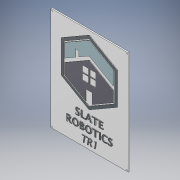
# Autodesk Inventor part: BP002b
Saved by Autodesk Inventor 2017 SP1 (Build 210196100, 196)
## iProperties
Created: 2017-12-18
Part Number: BP002b
Material: ABS Plastic
Document SubType Name: Modeling
Designer: Zach
Density: 1.06 g/cm^3
Appearance: CR White
Author: Zach
Autodesk Inventor part; units mm, degrees
ref_plane "YZ Plane" through (0, 0, 0) normal (1, 0, 0) x (0, 1, 0)
ref_plane "XZ Plane" through (0, 0, 0) normal (0, 1, 0) x (-1, 0, 0)
ref_plane "XY Plane" through (0, 0, 0) normal (0, 0, 1) x (1, 0, 0)
sketch "Sketch1" plane through (0, 0, 0) normal (0, 0, 1) x (1, 0, 0)
  line L0 (0, 0) -> (300, 0)
  line L1 (300, 0) -> (300, 400)
  line L2 (300, 400) -> (0, 400)
  line L3 (0, 400) -> (0, 0)
  line L4 (5, 5) -> (295, 5) construction
  line L5 (295, 5) -> (295, 395) construction
  line L6 (295, 395) -> (5, 395) construction
  line L7 (5, 395) -> (5, 5) construction
  circle A0 centre (5, 395) radius 2.5
  circle A1 centre (295, 395) radius 2.5
  circle A2 centre (295, 5) radius 2.5
  circle A3 centre (5, 5) radius 2.5
  dimension "d0" = 300
  dimension "d1" = 400
  dimension "d2" = 5
  dimension "d3" = 5
  dimension "d4" = 5
  dimension "d5" = 5
  dimension "d6" = 5
  constraints: 16 end point, 4 centre point, 4 coincident, 4 parallel, 2 perpendicular, 1 horizontal, 3 other
  measures "d0" distance of L2.end L1.end
  measures "d1" distance of L1.end L0.end
  measures "d2" distance between parallel lines of L3 L7
  measures "d3" diameter of A0
  measures "d4" diameter of A1
  measures "d5" diameter of A2
  measures "d6" diameter of A3
extrude "Extrusion1" add sketch "Sketch1" along normal blind 5
sketch "Sketch2" plane through (0, 0, 5) normal (0, 0, 1) x (1, 0, 0)
  line L0 (0, 135) -> (300, 135) construction
  line L1 (300, 135) -> (300, 0) construction
  line L2 (300, 0) -> (0, 0) construction
  line L3 (0, 0) -> (0, 135) construction
  line L4 (25, 385) -> (275, 385) construction
  line L5 (275, 385) -> (275, 135) construction
  line L6 (275, 135) -> (25, 135) construction
  line L7 (25, 135) -> (25, 385) construction
  line L8 (300, 400) -> (0, 400) projected
  line L9 (300, 0) -> (300, 400) projected
  line L10 (150, 385) -> (258.2532, 322.5)
  line L11 (258.2532, 322.5) -> (258.2532, 197.5)
  line L12 (258.2532, 197.5) -> (150, 135)
  line L13 (150, 135) -> (41.7468, 197.5)
  line L14 (41.7468, 197.5) -> (41.7468, 322.5)
  line L15 (41.7468, 322.5) -> (150, 385)
  line L16 (150, 373.2221) -> (248.0532, 316.611)
  line L17 (248.0532, 316.611) -> (248.0532, 203.389)
  line L18 (248.0532, 203.389) -> (150, 146.7779)
  line L19 (150, 146.7779) -> (51.9468, 203.389)
  line L20 (51.9468, 203.389) -> (51.9468, 316.611)
  line L21 (51.9468, 316.611) -> (150, 373.2221)
  line L22 (150, 368.3146) -> (243.8032, 314.1573) construction
  line L23 (243.8032, 314.1573) -> (243.8032, 205.8427) construction
  line L24 (243.8032, 205.8427) -> (150, 151.6854) construction
  line L25 (150, 151.6854) -> (56.1968, 205.8427) construction
  line L26 (56.1968, 205.8427) -> (56.1968, 314.1573) construction
  line L27 (56.1968, 314.1573) -> (150, 368.3146) construction
  line L28 (56.1968, 261.6573) -> (96.1968, 284.7513)
  line L29 (96.1968, 284.7513) -> (96.1968, 313.2513)
  line L30 (96.1968, 313.2513) -> (110.1968, 313.2513)
  line L31 (110.1968, 313.2513) -> (110.1968, 292.8342)
  line L32 (110.1968, 292.8342) -> (150, 315.8146)
  line L33 (150, 315.8146) -> (243.8032, 261.6573)
  line L34 (243.8032, 261.6573) -> (243.8032, 314.1573)
  line L35 (243.8032, 314.1573) -> (150, 368.3146)
  line L36 (150, 368.3146) -> (56.1968, 314.1573)
  line L37 (56.1968, 261.6573) -> (56.1968, 314.1573)
  line L38 (56.1968, 205.8427) -> (138, 158.6136)
  line L39 (138, 158.6136) -> (138, 198.6854)
  line L40 (138, 198.6854) -> (162, 198.6854)
  line L41 (162, 198.6854) -> (162, 158.6136)
  line L42 (162, 158.6136) -> (243.8032, 205.8427)
  line L43 (243.8032, 205.8427) -> (243.8032, 246.6573)
  line L44 (243.8032, 246.6573) -> (150, 300.8146)
  line L45 (150, 300.8146) -> (56.1968, 246.6573)
  line L46 (56.1968, 246.6573) -> (56.1968, 205.8427)
  line L47 (123.75, 272.6854) -> (176.25, 272.6854) construction
  line L48 (176.25, 272.6854) -> (176.25, 221.6854) construction
  line L49 (176.25, 221.6854) -> (123.75, 221.6854) construction
  line L50 (123.75, 221.6854) -> (123.75, 272.6854) construction
  line L51 (123.75, 221.6854) -> (147.75, 221.6854)
  line L52 (147.75, 221.6854) -> (147.75, 245.6854)
  line L53 (147.75, 245.6854) -> (123.75, 245.6854)
  line L54 (123.75, 245.6854) -> (123.75, 221.6854)
  line L55 (123.75, 272.6854) -> (147.75, 272.6854)
  line L56 (147.75, 272.6854) -> (147.75, 248.6854)
  line L57 (147.75, 248.6854) -> (123.75, 248.6854)
  line L58 (123.75, 248.6854) -> (123.75, 272.6854)
  line L59 (176.25, 272.6854) -> (152.25, 272.6854)
  line L60 (152.25, 272.6854) -> (152.25, 248.6854)
  line L61 (152.25, 248.6854) -> (176.25, 248.6854)
  line L62 (176.25, 248.6854) -> (176.25, 272.6854)
  line L63 (176.25, 221.6854) -> (152.25, 221.6854)
  line L64 (152.25, 221.6854) -> (152.25, 245.6854)
  line L65 (152.25, 245.6854) -> (176.25, 245.6854)
  line L66 (176.25, 245.6854) -> (176.25, 221.6854)
  line L67 (96.7483, 94.8958) -> (96.7483, 99.1804)
  spline S0 degree 2 poles (96.7483, 99.1804) (99.6748, 97.9563) (102.5631, 97.4781) (103.7682, 97.4781) knots 0 0 0 1 2 2 2
  spline S1 degree 2 poles (103.7682, 97.4781) (105.9487, 97.4781) (108.1102, 99.4291) (108.1102, 100.8063) knots 0 0 0 1 2 2 2
  spline S2 degree 2 poles (108.1102, 100.8063) (108.1102, 101.8583) (107.5172, 102.7) knots 0 0 0 1 1 1
  spline S3 degree 2 poles (107.5172, 102.7) (106.9051, 103.5224) (104.5524, 104.8423) knots 0 0 0 1 1 1
  line L68 (104.5524, 104.8423) -> (102.8692, 105.7795)
  spline S4 degree 2 poles (102.8692, 105.7795) (99.254, 107.7879) (97.9916, 109.4903) knots 0 0 0 1 1 1
  spline S5 degree 2 poles (97.9916, 109.4903) (96.6909, 111.1927) (96.6909, 113.4306) knots 0 0 0 1 1 1
  spline S6 degree 2 poles (96.6909, 113.4306) (96.6909, 116.2615) (101.0138, 120.2784) (105.0497, 120.2784) knots 0 0 0 1 2 2 2
  spline S7 degree 2 poles (105.0497, 120.2784) (108.0719, 120.2784) (111.8592, 119.4176) knots 0 0 0 1 1 1
  line L69 (111.8592, 119.4176) -> (111.8592, 115.4199)
  spline S8 degree 2 poles (111.8592, 115.4199) (107.9763, 116.8545) (105.7001, 116.8545) knots 0 0 0 1 1 1
  spline S9 degree 2 poles (105.7001, 116.8545) (103.8064, 116.8545) (101.8363, 115.2095) (101.8363, 114.0618) knots 0 0 0 1 2 2 2
  spline S10 degree 2 poles (101.8363, 114.0618) (101.8363, 113.182) (102.4484, 112.436) knots 0 0 0 1 1 1
  spline S11 degree 2 poles (102.4484, 112.436) (103.0222, 111.6709) (105.3749, 110.3511) knots 0 0 0 1 1 1
  line L70 (105.3749, 110.3511) -> (107.1729, 109.3564)
  spline S12 degree 2 poles (107.1729, 109.3564) (111.3236, 107.042) (112.4522, 105.3396) knots 0 0 0 1 1 1
  spline S13 degree 2 poles (112.4522, 105.3396) (113.5807, 103.6181) (113.5807, 101.4758) knots 0 0 0 1 1 1
  spline S14 degree 2 poles (113.5807, 101.4758) (113.5807, 98.3962) (108.8944, 94.0542) (103.7873, 94.0542) knots 0 0 0 1 2 2 2
  spline S15 degree 2 poles (103.7873, 94.0542) (100.7651, 94.0542) (96.7483, 94.8958) knots 0 0 0 1 1 1
  line L71 (117.9036, 94.6663) -> (117.9036, 119.6663)
  line L72 (117.9036, 119.6663) -> (123.1064, 119.6663)
  line L73 (123.1064, 119.6663) -> (123.1064, 98.2049)
  line L74 (123.1064, 98.2049) -> (134.2578, 98.2049)
  line L75 (134.2578, 98.2049) -> (134.2578, 94.6663)
  line L76 (134.2578, 94.6663) -> (117.9036, 94.6663)
  line L77 (135.2716, 94.6663) -> (144.9694, 119.6663)
  line L78 (144.9694, 119.6663) -> (150.1913, 119.6663)
  line L79 (150.1913, 119.6663) -> (159.9273, 94.6663)
  line L80 (159.9273, 94.6663) -> (154.5907, 94.6663)
  line L81 (154.5907, 94.6663) -> (151.9893, 101.3419)
  line L82 (151.9893, 101.3419) -> (141.6603, 101.3419)
  line L83 (141.6603, 101.3419) -> (139.0589, 94.6663)
  line L84 (139.0589, 94.6663) -> (135.2716, 94.6663)
  line L85 (142.9419, 104.6701) -> (150.6886, 104.6701)
  line L86 (150.6886, 104.6701) -> (146.8248, 114.6357)
  line L87 (146.8248, 114.6357) -> (142.9419, 104.6701)
  line L88 (169.6825, 94.6663) -> (169.6825, 116.2233)
  line L89 (169.6825, 116.2233) -> (160.7307, 116.2233)
  line L90 (160.7307, 116.2233) -> (160.7307, 119.6663)
  line L91 (160.7307, 119.6663) -> (183.837, 119.6663)
  line L92 (183.837, 119.6663) -> (183.837, 116.2233)
  line L93 (183.837, 116.2233) -> (174.8852, 116.2233)
  line L94 (174.8852, 116.2233) -> (174.8852, 94.6663)
  line L95 (174.8852, 94.6663) -> (169.6825, 94.6663)
  line L96 (187.3183, 94.6663) -> (187.3183, 119.6663)
  line L97 (187.3183, 119.6663) -> (203.3282, 119.6663)
  line L98 (203.3282, 119.6663) -> (203.3282, 116.2233)
  line L99 (203.3282, 116.2233) -> (192.521, 116.2233)
  line L100 (192.521, 116.2233) -> (192.521, 109.2608)
  line L101 (192.521, 109.2608) -> (201.4537, 109.2608)
  line L102 (201.4537, 109.2608) -> (201.4537, 105.8178)
  line L103 (201.4537, 105.8178) -> (192.521, 105.8178)
  line L104 (192.521, 105.8178) -> (192.521, 98.2049)
  line L105 (192.521, 98.2049) -> (204.1316, 98.2049)
  line L106 (204.1316, 98.2049) -> (204.1316, 94.6663)
  line L107 (204.1316, 94.6663) -> (187.3183, 94.6663)
  line L108 (61.9836, 54.7098) -> (61.9836, 79.7098)
  line L109 (61.9836, 79.7098) -> (71.337, 79.7098)
  spline S16 degree 2 poles (71.337, 79.7098) (74.2062, 79.7098) (77.2093, 78.2752) (78.9499, 75.3486) (78.9499, 73.5124) knots 0 0 0 1 2 3 3 3
  spline S17 degree 2 poles (78.9499, 73.5124) (78.9499, 71.3127) (76.425, 67.4106) (74.1106, 66.3777) knots 0 0 0 1 2 2 2
  line L110 (74.1106, 66.3777) -> (82.2781, 54.7098)
  line L111 (82.2781, 54.7098) -> (75.9468, 54.7098)
  line L112 (75.9468, 54.7098) -> (69.7303, 64.924)
  line L113 (69.7303, 64.924) -> (66.8803, 64.924)
  line L114 (66.8803, 64.924) -> (66.8803, 54.7098)
  line L115 (66.8803, 54.7098) -> (61.9836, 54.7098)
  line L116 (66.8803, 68.3479) -> (68.0662, 68.3479)
  spline S18 degree 2 poles (68.0662, 68.3479) (71.2797, 68.3479) (73.7471, 71.1597) (73.7471, 72.9385) knots 0 0 0 1 2 2 2
  spline S19 degree 2 poles (73.7471, 72.9385) (73.7471, 74.4688) (71.7578, 76.2859) (68.6974, 76.2859) knots 0 0 0 1 2 2 2
  line L117 (68.6974, 76.2859) -> (66.8803, 76.2859)
  line L118 (66.8803, 76.2859) -> (66.8803, 68.3479)
  spline S20 degree 2 poles (96.9683, 54.0977) (93.0662, 54.0977) (87.2896, 57.3303) (84.2865, 63.3747) (84.2865, 67.2193) knots 0 0 0 1 2 3 3 3
  spline S21 degree 2 poles (84.2865, 67.2193) (84.2865, 71.0258) (87.2896, 77.1084) (93.1044, 80.3219) (96.9683, 80.3219) knots 0 0 0 1 2 3 3 3
  spline S22 degree 2 poles (96.9683, 80.3219) (100.8129, 80.3219) (106.6278, 77.1084) (109.6308, 71.0258) (109.6308, 67.2193) knots 0 0 0 1 2 3 3 3
  spline S23 degree 2 poles (109.6308, 67.2193) (109.6308, 63.3747) (106.6278, 57.3303) (100.8703, 54.0977) (96.9683, 54.0977) knots 0 0 0 1 2 3 3 3
  spline S24 degree 2 poles (96.9683, 57.5216) (100.5834, 57.5216) (104.1029, 63.4129) (104.1029, 67.2193) knots 0 0 0 1 2 2 2
  spline S25 degree 2 poles (104.1029, 67.2193) (104.1029, 71.0449) (100.5643, 76.898) (96.9683, 76.898) knots 0 0 0 1 2 2 2
  spline S26 degree 2 poles (96.9683, 76.898) (93.3531, 76.898) (89.8145, 71.0449) (89.8145, 67.2193) knots 0 0 0 1 2 2 2
  spline S27 degree 2 poles (89.8145, 67.2193) (89.8145, 63.4129) (93.334, 57.5216) (96.9683, 57.5216) knots 0 0 0 1 2 2 2
  line L119 (114.298, 54.7098) -> (114.298, 79.7098)
  line L120 (114.298, 79.7098) -> (122.7334, 79.7098)
  spline S28 degree 2 poles (122.7334, 79.7098) (125.7938, 79.7098) (128.7204, 78.3326) (130.3845, 75.6547) (130.3845, 74.1436) knots 0 0 0 1 2 3 3 3
  spline S29 degree 2 poles (130.3845, 74.1436) (130.3845, 72.2691) (127.7831, 68.8261) (124.4166, 67.774) knots 0 0 0 1 2 2 2
  spline S30 degree 2 poles (124.4166, 67.774) (127.0945, 67.1046) (129.9254, 65.1535) (131.3982, 62.4374) (131.3982, 60.888) knots 0 0 0 1 2 3 3 3
  spline S31 degree 2 poles (131.3982, 60.888) (131.3982, 59.2048) (129.6767, 56.2783) (126.6546, 54.7098) (123.5176, 54.7098) knots 0 0 0 1 2 3 3 3
  line L121 (123.5176, 54.7098) -> (114.298, 54.7098)
  line L122 (119.2904, 58.2484) -> (120.285, 58.2484)
  spline S32 degree 2 poles (120.285, 58.2484) (123.0012, 58.2484) (124.9713, 58.9561) (125.966, 60.5437) (125.966, 61.5193) knots 0 0 0 1 2 3 3 3
  spline S33 degree 2 poles (125.966, 61.5193) (125.966, 63.3747) (122.6951, 65.9569) (120.1894, 65.9569) knots 0 0 0 1 2 2 2
  line L123 (120.1894, 65.9569) -> (119.2904, 65.9569)
  line L124 (119.2904, 65.9569) -> (119.2904, 58.2484)
  line L125 (119.2904, 69.3043) -> (120.3998, 69.3043)
  spline S34 degree 2 poles (120.3998, 69.3043) (122.7716, 69.3043) (125.1052, 71.657) (125.1052, 73.3402) knots 0 0 0 1 2 2 2
  spline S35 degree 2 poles (125.1052, 73.3402) (125.1052, 74.2392) (124.4166, 75.5591) (122.676, 76.2859) (120.2276, 76.2859) knots 0 0 0 1 2 3 3 3
  line L126 (120.2276, 76.2859) -> (119.2904, 76.2859)
  line L127 (119.2904, 76.2859) -> (119.2904, 69.3043)
  spline S36 degree 2 poles (147.2169, 54.0977) (143.3148, 54.0977) (137.5383, 57.3303) (134.5352, 63.3747) (134.5352, 67.2193) knots 0 0 0 1 2 3 3 3
  spline S37 degree 2 poles (134.5352, 67.2193) (134.5352, 71.0258) (137.5383, 77.1084) (143.3531, 80.3219) (147.2169, 80.3219) knots 0 0 0 1 2 3 3 3
  spline S38 degree 2 poles (147.2169, 80.3219) (151.0616, 80.3219) (156.8764, 77.1084) (159.8795, 71.0258) (159.8795, 67.2193) knots 0 0 0 1 2 3 3 3
  spline S39 degree 2 poles (159.8795, 67.2193) (159.8795, 63.3747) (156.8764, 57.3303) (151.119, 54.0977) (147.2169, 54.0977) knots 0 0 0 1 2 3 3 3
  spline S40 degree 2 poles (147.2169, 57.5216) (150.8321, 57.5216) (154.3516, 63.4129) (154.3516, 67.2193) knots 0 0 0 1 2 2 2
  spline S41 degree 2 poles (154.3516, 67.2193) (154.3516, 71.0449) (150.8129, 76.898) (147.2169, 76.898) knots 0 0 0 1 2 2 2
  spline S42 degree 2 poles (147.2169, 76.898) (143.6018, 76.898) (140.0631, 71.0449) (140.0631, 67.2193) knots 0 0 0 1 2 2 2
  spline S43 degree 2 poles (140.0631, 67.2193) (140.0631, 63.4129) (143.5826, 57.5216) (147.2169, 57.5216) knots 0 0 0 1 2 2 2
  line L128 (170.7632, 54.7098) -> (170.7632, 76.2668)
  line L129 (170.7632, 76.2668) -> (161.8114, 76.2668)
  line L130 (161.8114, 76.2668) -> (161.8114, 79.7098)
  line L131 (161.8114, 79.7098) -> (184.9178, 79.7098)
  line L132 (184.9178, 79.7098) -> (184.9178, 76.2668)
  line L133 (184.9178, 76.2668) -> (175.966, 76.2668)
  line L134 (175.966, 76.2668) -> (175.966, 54.7098)
  line L135 (175.966, 54.7098) -> (170.7632, 54.7098)
  line L136 (188.399, 54.7098) -> (188.399, 79.7098)
  line L137 (188.399, 79.7098) -> (193.6018, 79.7098)
  line L138 (193.6018, 79.7098) -> (193.6018, 54.7098)
  line L139 (193.6018, 54.7098) -> (188.399, 54.7098)
  spline S44 degree 2 poles (219.979, 55.7044) (218.334, 54.9776) (215.9047, 54.442) (212.8252, 54.0977) (211.3141, 54.0977) knots 0 0 0 1 2 3 3 3
  spline S45 degree 2 poles (211.3141, 54.0977) (204.7533, 54.0977) (198.3072, 61.481) (198.3072, 67.2193) knots 0 0 0 1 2 2 2
  spline S46 degree 2 poles (198.3072, 67.2193) (198.3072, 72.9577) (204.7341, 80.3219) (211.6393, 80.3219) knots 0 0 0 1 2 2 2
  spline S47 degree 2 poles (211.6393, 80.3219) (215.7135, 80.3219) (219.7494, 79.3655) knots 0 0 0 1 1 1
  line L140 (219.7494, 79.3655) -> (219.7494, 75.2913)
  spline S48 degree 2 poles (219.7494, 75.2913) (217.7984, 75.9607) (215.3309, 76.592) (213.1312, 76.898) (212.0218, 76.898) knots 0 0 0 1 2 3 3 3
  spline S49 degree 2 poles (212.0218, 76.898) (207.7181, 76.898) (203.8351, 71.3701) (203.8351, 67.2767) knots 0 0 0 1 2 2 2
  spline S50 degree 2 poles (203.8351, 67.2767) (203.8351, 62.9921) (208.2345, 57.6937) (212.5956, 57.6937) knots 0 0 0 1 2 2 2
  spline S51 degree 2 poles (212.5956, 57.6937) (216.2299, 57.6937) (219.979, 59.53) knots 0 0 0 1 1 1
  line L141 (219.979, 59.53) -> (219.979, 55.7044)
  line L142 (223.0968, 54.9393) -> (223.0968, 59.2239)
  spline S52 degree 2 poles (223.0968, 59.2239) (226.0233, 57.9998) (228.9116, 57.5216) (230.1167, 57.5216) knots 0 0 0 1 2 2 2
  spline S53 degree 2 poles (230.1167, 57.5216) (232.2973, 57.5216) (234.4587, 59.4726) (234.4587, 60.8498) knots 0 0 0 1 2 2 2
  spline S54 degree 2 poles (234.4587, 60.8498) (234.4587, 61.9018) (233.8657, 62.7434) knots 0 0 0 1 1 1
  spline S55 degree 2 poles (233.8657, 62.7434) (233.2536, 63.5659) (230.9009, 64.8858) knots 0 0 0 1 1 1
  line L143 (230.9009, 64.8858) -> (229.2177, 65.823)
  spline S56 degree 2 poles (229.2177, 65.823) (225.6025, 67.8314) (224.3401, 69.5338) knots 0 0 0 1 1 1
  spline S57 degree 2 poles (224.3401, 69.5338) (223.0394, 71.2362) (223.0394, 73.4741) knots 0 0 0 1 1 1
  spline S58 degree 2 poles (223.0394, 73.4741) (223.0394, 76.305) (227.3623, 80.3219) (231.3982, 80.3219) knots 0 0 0 1 2 2 2
  spline S59 degree 2 poles (231.3982, 80.3219) (234.4204, 80.3219) (238.2077, 79.4611) knots 0 0 0 1 1 1
  line L144 (238.2077, 79.4611) -> (238.2077, 75.4634)
  spline S60 degree 2 poles (238.2077, 75.4634) (234.3248, 76.898) (232.0486, 76.898) knots 0 0 0 1 1 1
  spline S61 degree 2 poles (232.0486, 76.898) (230.1549, 76.898) (228.1848, 75.253) (228.1848, 74.1053) knots 0 0 0 1 2 2 2
  spline S62 degree 2 poles (228.1848, 74.1053) (228.1848, 73.2255) (228.7969, 72.4795) knots 0 0 0 1 1 1
  spline S63 degree 2 poles (228.7969, 72.4795) (229.3707, 71.7144) (231.7234, 70.3946) knots 0 0 0 1 1 1
  line L145 (231.7234, 70.3946) -> (233.5214, 69.3999)
  spline S64 degree 2 poles (233.5214, 69.3999) (237.6722, 67.0854) (238.8007, 65.3831) knots 0 0 0 1 1 1
  spline S65 degree 2 poles (238.8007, 65.3831) (239.9292, 63.6616) (239.9292, 61.5193) knots 0 0 0 1 1 1
  spline S66 degree 2 poles (239.9292, 61.5193) (239.9292, 58.4397) (235.2429, 54.0977) (230.1358, 54.0977) knots 0 0 0 1 2 2 2
  spline S67 degree 2 poles (230.1358, 54.0977) (227.1136, 54.0977) (223.0968, 54.9393) knots 0 0 0 1 1 1
  line L146 (126.3462, 14.7216) -> (130.8077, 37.0678)
  line L147 (130.8077, 37.0678) -> (121.9231, 37.0678)
  line L148 (121.9231, 37.0678) -> (122.4423, 39.7216)
  line L149 (122.4423, 39.7216) -> (143.7308, 39.7216)
  line L150 (143.7308, 39.7216) -> (143.1923, 37.0678)
  line L151 (143.1923, 37.0678) -> (134.3269, 37.0678)
  line L152 (134.3269, 37.0678) -> (129.8846, 14.7216)
  line L153 (129.8846, 14.7216) -> (126.3462, 14.7216)
  line L154 (142.1346, 14.7216) -> (147.1154, 39.7216)
  line L155 (147.1154, 39.7216) -> (154.6538, 39.7216)
  spline S68 degree 2 poles (154.6538, 39.7216) (156.6346, 39.7216) (159.3462, 39.0485) (161.1346, 36.6255) (161.1346, 34.8755) knots 0 0 0 1 2 3 3 3
  spline S69 degree 2 poles (161.1346, 34.8755) (161.1346, 32.337) (157.5192, 27.837) (154.4423, 26.6639) knots 0 0 0 1 2 2 2
  line L156 (154.4423, 26.6639) -> (160.3846, 14.7216)
  line L157 (160.3846, 14.7216) -> (156.4615, 14.7216)
  line L158 (156.4615, 14.7216) -> (151.2115, 25.7793)
  line L159 (151.2115, 25.7793) -> (147.8654, 25.7793)
  line L160 (147.8654, 25.7793) -> (145.6731, 14.7216)
  line L161 (145.6731, 14.7216) -> (142.1346, 14.7216)
  line L162 (148.3846, 28.3947) -> (150.3462, 28.3947)
  spline S70 degree 2 poles (150.3462, 28.3947) (152.4423, 28.3947) (155.5385, 29.9716) (157.3654, 32.9716) (157.3654, 34.4716) knots 0 0 0 1 2 3 3 3
  spline S71 degree 2 poles (157.3654, 34.4716) (157.3654, 35.7601) (155.4038, 37.0678) (152.3654, 37.0678) knots 0 0 0 1 2 2 2
  line L163 (152.3654, 37.0678) -> (150.1154, 37.0678)
  line L164 (150.1154, 37.0678) -> (148.3846, 28.3947)
  line L165 (169.8269, 14.7216) -> (174.3077, 37.1832)
  line L166 (174.3077, 37.1832) -> (170.4038, 37.1832)
  line L167 (170.4038, 37.1832) -> (170.8269, 39.2601)
  line L168 (170.8269, 39.2601) -> (178.2115, 39.9332)
  line L169 (178.2115, 39.9332) -> (173.1538, 14.7216)
  line L170 (173.1538, 14.7216) -> (169.8269, 14.7216)
  point P0 (150, 260)
  point P1 (150, 198.6854)
  point P2 (150, 272.6854)
  dimension "d21" = 15
  dimension "d27" = 250
  dimension "d31" = 10.2
  dimension "d32" = 4.25
  dimension "d41" = 52.5
  dimension "d42" = 40
  dimension "d43" = 14
  dimension "d44" = 28.5
  dimension "d46" = 15
  dimension "d48" = 24
  dimension "d49" = 47
  dimension "d50" = 23
  dimension "d52" = 51
  dimension "d53" = 52.5
  dimension "d54" = 24
  dimension "d55" = 24
  dimension "d56" = 24
  dimension "d57" = 24
  dimension "d58" = 24
  dimension "d59" = 24
  dimension "d60" = 24
  dimension "d61" = 24
  constraints: 114 end point, 15 parallel, 9 perpendicular, 8 point on line, 5 horizontal, 5 midpoint, 5 vertical alignment, 4 collinear, 2 coincident, 2 vertical, 27 other
  measures "d21" distance between parallel lines of L8 L4
  measures "d27" distance of L4.start L4.end
  measures "d31" distance between parallel lines of L15 L21
  measures "d32" distance between parallel lines of L21 L27
  measures "d41" distance of L28.start L26.end
  measures "d42" distance between parallel lines of L26 L29
  measures "d43" distance of L29.end L30.end
  measures "d44" distance of L28.end L29.end
  measures "d46" distance of L32.end L44.end
  measures "d48" distance between parallel lines of L41 L39
  measures "d49" distance from line of L24.end L40
  measures "d50" distance between parallel lines of L40 L49
  measures "d52" distance of L49.end L47.start
  measures "d53" distance of L47.start L47.end
  measures "d54" distance of L53.end L52.end
  measures "d55" distance of L52.end L51.end
  measures "d56" distance of L56.end L57.end
  measures "d57" distance of L55.end L56.end
  measures "d58" distance of L61.end L60.end
  measures "d59" distance of L60.end L59.end
  measures "d60" distance of L64.end L65.end
  measures "d61" distance of L63.end L64.end
extrude "Extrusion2" add sketch "Sketch2" along normal blind 2
body "Solid1"
